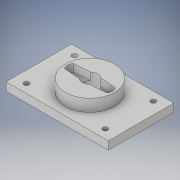
# Autodesk Inventor part: base
Saved by Autodesk Inventor 2017 (Build 210142000, 142)
## iProperties
Created: 2017-03-11
Part Number: base
Material: Generic
Document SubType Name: Modeling
Designer: Naga
Density: 1 g/cm^3
Appearance: Default
Author: Naga
Autodesk Inventor part; units mm, degrees
ref_plane "YZ Plane" through (0, 0, 0) normal (1, 0, 0) x (0, 1, 0)
ref_plane "XZ Plane" through (0, 0, 0) normal (0, 1, 0) x (-1, 0, 0)
ref_plane "XY Plane" through (0, 0, 0) normal (0, 0, 1) x (1, 0, 0)
sketch "Sketch1" plane through (0, 0, 0) normal (0, 1, 0) x (-1, 0, 0)
  line L0 (0, 0) -> (50, 0)
  line L1 (50, 0) -> (50, -32)
  line L2 (50, -32) -> (0, -32)
  line L3 (0, -32) -> (0, 0)
  line L4 (0, -27.752) -> (5.747, -27.752)
  circle A0 centre (5.747, -27.752) radius 1.25
  line L5 (25, 0) -> (25, -16) construction
  line L6 (25, -16) -> (0, -16) construction
  circle A1 centre (5.747, -4.248) radius 1.25
  circle A2 centre (44.253, -27.752) radius 1.25
  circle A3 centre (44.253, -4.248) radius 1.25
  circle A4 centre (25, -16) radius 3.75
  dimension "d0" = 50
  dimension "d1" = 32
  dimension "d2" = 5.747
  dimension "d3" = 4.248
  dimension "d4" = 2.5
  dimension "d5" = 7.5
  constraints: 14 end point, 5 centre point, 3 symmetric about line, 2 coincident, 2 horizontal, 2 midpoint, 2 parallel, 1 perpendicular, 1 point on line, 1 vertical, 3 other
  measures "d0" distance of L1.end L2.end
  measures "d1" distance of L0.end L1.end
  measures "d2" distance of L4.start L4.end
  measures "d3" distance between parallel lines of L2 L4
  measures "d4" diameter of A0
  measures "d5" diameter of A4
extrude "Extrusion1" add sketch "Sketch1" along normal blind 4
sketch "Sketch2" plane through (0, 4, 0) normal (0, 1, 0) x (1, 0, 0)
  circle A0 centre (-25, 16) radius 3.75 projected
  circle A1 centre (-25, 16) radius 12
  line L0 (-25, 16) -> (-32, 16)
  line L1 (-25, 16) -> (-18, 16)
  circle A2 centre (-32, 16) radius 0.75
  circle A3 centre (-18, 16) radius 0.75
  point P0 (0, 0)
  dimension "d8" = 24
  dimension "d9" = 7
  dimension "d10" = 7
  dimension "d11" = 1.5
  dimension "d12" = 1.5
  constraints: 4 end point, 3 centre point, 3 coincident, 2 horizontal
  measures "d8" diameter of A1
  measures "d9" distance of L0.start L0.end
  measures "d10" distance of L0.start L1.end
  measures "d11" diameter of A2
  measures "d12" diameter of A3
extrude "Extrusion2" add sketch "Sketch2" along normal blind 2.325
sketch "Sketch3" plane through (-25, 6.325, -16) normal (0, 1, 0) x (1, 0, 0)
  circle A0 centre (0, 0) radius 12 projected
  circle A1 centre (0, 0) radius 3.75 projected
  circle A2 centre (-7, 0) radius 0.75 projected
  circle A3 centre (7, 0) radius 0.75 projected
  line L0 (-7, 0) -> (-7.5625, 0)
  line L1 (-7, 0) -> (-7, -2.877)
  line L2 (-7, 0) -> (-10.333, 0)
  line L3 (-10.333, 2.1388) -> (-10.333, 2.277)
  line L4 (-10.333, -2.1388) -> (-10.333, -2.277)
  line L5 (-10.333, -2.1388) -> (-10.005, -2.1388)
  line L6 (-10.333, -2.1388) -> (-2.5151, -2.7815)
  line L7 (-10.333, -2.1388) -> (-2.4887, -2.1388) construction
  line L8 (0, 0) -> (0, 2.5608)
  line L9 (-10.333, 2.1388) -> (-2.5151, 2.7815)
  arc A4 (-5.1785, -2.5625) -> (-4.792, -2.1388) centre (-7.5625, 0) ccw
  arc A5 (-10.333, 2.1388) -> (-10.333, -2.1388) centre (-7.5625, 0) ccw
  line L10 (10.333, -2.1388) -> (2.5151, -2.7815)
  line L11 (10.333, 2.1388) -> (2.5151, 2.7815)
  arc A6 (10.333, -2.1388) -> (10.333, 2.1388) centre (7.5625, 0) ccw
  arc A7 (-3.0803, -2.1388) -> (2.5151, -2.7815) centre (0, 0) ccw
  arc A8 (2.5151, 2.7815) -> (-2.5151, 2.7815) centre (0, 0) ccw
  point P0 (25, -16)
  dimension "d15" = 0.5625
  dimension "d17" = 2.877
  dimension "d18" = 3.333
  dimension "d20" = 2.277
  dimension "d21" = 4.7
  constraints: 24 end point, 11 point on circle, 8 symmetric about line, 5 centre point, 4 point on line, 3 horizontal, 3 vertical, 2 coincident, 1 equal length, 3 other
  measures "d15" distance of L0.start L0.end
  measures "d17" distance of L0.start L1.end
  measures "d18" distance of L0.start L2.end
  measures "d20" distance of L2.end L3.end
  measures "d21" angle of L6 L7
extrude "Extrusion3" add sketch "Sketch3" along normal blind 3.675 contours A0
body "Solid1"
